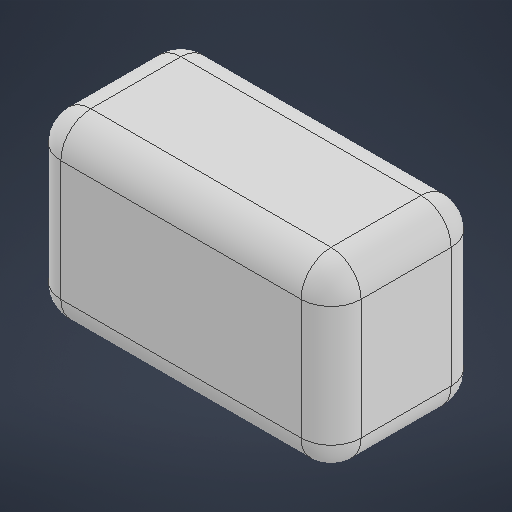
# Autodesk Inventor part: Battery
Saved by Autodesk Inventor 2026 (Build 300175050, 175E)
## iProperties
Created: 2026-07-07
Part Number: Battery
Material: 一般
Document SubType Name: Modeling
Designer: hanaj
Density: 1 g/cm^3
Appearance: 既定
Author: hanaj
Autodesk Inventor part; units mm, degrees
ref_plane "YZ Plane" through (0, 0, 0) normal (1, 0, 0) x (0, 1, 0)
ref_plane "XZ Plane" through (0, 0, 0) normal (0, 1, 0) x (-1, 0, 0)
ref_plane "XY Plane" through (0, 0, 0) normal (0, 0, 1) x (1, 0, 0)
sketch "スケッチ1" plane through (0, 0, 0) normal (0, 0, 1) x (1, 0, 0)
  line L0 (0, 0) -> (30, 0)
  line L1 (30, 0) -> (30, 18)
  line L2 (30, 18) -> (0, 18)
  line L3 (0, 18) -> (0, 0)
  dimension "d0" = 30
  dimension "d1" = 18
  constraints: 8 end point, 2 parallel, 1 horizontal, 1 perpendicular
  measures "d0" distance of L2.end L1.end
  measures "d1" distance of L1.end L0.end
extrude "押し出し1" add sketch "スケッチ1" along normal blind 15
fillet "フィレット1" radius 3 12 edges at (0, 18, 7.5) (0, 9, 15) (0, 9, 0) (0, 0, 7.5) (30, 9, 15) (30, 9, 0) (30, 18, 7.5) (15, 0, 15) (30, 0, 7.5) (15, 0, 0) (15, 18, 15) (15, 18, 0)
